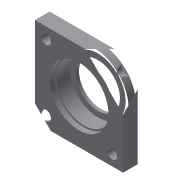
# Autodesk Inventor part: Module Top Cap
Saved by Autodesk Inventor 2014 SP1 (Build 180222100, 222)
## iProperties
Created: 2014-05-05
Part Number: Module Top Cap
Material: Generic
Document SubType Name: Modeling
Designer: Rauhul Varma
Density: 1 g/cm^3
Appearance: Default
Author: Rauhul Varma
Autodesk Inventor part; units mm, degrees
ref_plane "YZ Plane" through (0, 0, 0) normal (1, 0, 0) x (0, 1, 0)
ref_plane "XZ Plane" through (0, 0, 0) normal (0, 1, 0) x (-1, 0, 0)
ref_plane "XY Plane" through (0, 0, 0) normal (0, 0, 1) x (1, 0, 0)
sketch "Sketch1" plane through (0, 0, 0) normal (0, 0, 1) x (1, 0, 0)
  line L0 (-19.05, -19.05) -> (19.05, -19.05)
  line L1 (19.05, -19.05) -> (19.05, 19.05)
  line L2 (19.05, 19.05) -> (-19.05, 19.05)
  line L3 (-19.05, 19.05) -> (-19.05, -19.05)
  line L4 (-19.05, -19.05) -> (19.05, 19.05) construction
  line L5 (19.05, -19.05) -> (-19.05, 19.05) construction
  line L6 (14.2875, -14.2875) -> (-14.2875, -14.2875) construction
  line L7 (-14.2875, -14.2875) -> (-14.2875, 14.2875) construction
  line L8 (-14.2875, 14.2875) -> (14.2875, 14.2875) construction
  line L9 (14.2875, 14.2875) -> (14.2875, -14.2875) construction
  line L10 (14.2875, -14.2875) -> (-14.2875, 14.2875) construction
  line L11 (-14.2875, -14.2875) -> (14.2875, 14.2875) construction
  circle A0 centre (0, 0) radius 12.7
  circle A1 centre (0, 0) radius 12
  circle A2 centre (0, 0) radius 9.525
  dimension "d0" = 38.1
  dimension "d1" = 38.1
  dimension "d3" = 25.4
  dimension "d4" = 24
  dimension "d5" = 19.05
  dimension "d20" = 28.575
  constraints: 24 end point, 7 coincident, 5 midpoint, 4 parallel, 3 centre point, 2 horizontal, 2 perpendicular, 1 point on line
  measures "d0" distance of L2.end L1.end
  measures "d1" distance of L1.end L0.end
  measures "d3" diameter of A0
  measures "d4" diameter of A1
  measures "d5" diameter of A2
  measures "d20" distance of L6.end L7.end
extrude "Extrusion1" add sketch "Sketch1" against normal blind 9.525 contours L3 L2 L1 L0 | A0 | A1
extrude "Extrusion2" cut sketch "Sketch1" against normal blind 2.1906 contours A0
extrude "Extrusion3" cut sketch "Sketch1" against normal blind 8.1906 contours A1
hole "Hole1" at (-14.2875, 14.2875, 0) at (14.2875, 14.2875, 0) at (14.2875, -14.2875, 0) at (-14.2875, -14.2875, 0) direction (0, 0, -1) diameter 4.318 end through all clearance for "Socket Head Cap Screw" size "#8" standard "Ansi Unified Screw Threads"
sketch "Sketch2" plane through (0, 0, -9.525) normal (0, 0, -1) x (-1, 0, 0)
  line L0 (-19.05, -19.05) -> (19.05, -19.05) projected
  line L1 (19.05, -19.05) -> (19.05, 19.05) projected
  line L2 (19.05, 19.05) -> (-19.05, 19.05) projected
  line L3 (-19.05, 19.05) -> (-19.05, -19.05) projected
  circle A0 centre (-14.2875, -14.2875) radius 2.159 projected
  circle A1 centre (14.2875, 14.2875) radius 2.159 projected
  circle A2 centre (-14.2875, 14.2875) radius 2.159 projected
  circle A3 centre (14.2875, -14.2875) radius 2.159 projected
  circle A4 centre (0, 0) radius 9.525 projected
  circle A5 centre (-14.2875, 14.2875) radius 3.429 construction
  circle A6 centre (0, 0) radius 12 construction
  circle A7 centre (0, 0) radius 15.0812
  dimension "d21" = 6.858
  dimension "d22" = 24
  dimension "d23" = 30.1625
  constraints: 3 centre point, 3 coincident
  measures "d21" diameter of A5
  measures "d22" diameter of A6
  measures "d23" diameter of A7
extrude "Extrusion4" cut sketch "Sketch2" against normal blind 3.175 contours L3 L2 L1 L0
equation "\"d1\" = d0"
body "Solid1"
